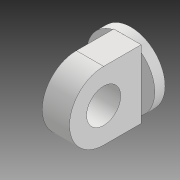
# Autodesk Inventor part: Link3
Saved by Autodesk Inventor 2020 (Build 240168000, 168)
## iProperties
Created: 2021-03-25
Part Number: Link3
Material: Generic
Document SubType Name: Modeling
Designer: DDeGo
Density: 1 g/cm^3
Appearance: Default
Author: DDeGo
Autodesk Inventor part; units mm, degrees
ref_plane "YZ Plane" through (0, 0, 0) normal (1, 0, 0) x (0, 1, 0)
ref_plane "XZ Plane" through (0, 0, 0) normal (0, 1, 0) x (-1, 0, 0)
ref_plane "XY Plane" through (0, 0, 0) normal (0, 0, 1) x (1, 0, 0)
sketch "Sketch1" plane through (0, 0, 0) normal (1, 0, 0) x (0, 1, 0)
  circle A0 centre (0, 0) radius 25
  arc A1 (50, 0) -> (-50, 0) centre (0, 0) ccw
  line L0 (50, 0) -> (-50, 0) construction
  line L1 (-50, 0) -> (-50, -55)
  line L2 (-50, -55) -> (50, -55)
  line L3 (50, -55) -> (50, 0)
  dimension "d0" = 50
  dimension "d1" = 100
  dimension "d4" = 55
  constraints: 8 end point, 2 centre point, 2 coincident, 2 parallel, 2 point on circle, 1 horizontal, 1 midpoint, 1 perpendicular
  measures "d0" diameter of A0
  measures "d1" diameter of A1
  measures "d4" distance from line of L2 point (0, 0)
extrude "Extrusion1" add sketch "Sketch1" along normal mid plane 40
sketch "Sketch2" plane through (-20, -50, -55) normal (0, 0, -1) x (-1, 0, 0)
  line L0 (-20, 50) -> (0, 50) construction
  circle A0 centre (0, 50) radius 50
  dimension "d5" = 100
  dimension "d9" = 20
  constraints: 2 end point, 1 centre point, 1 coincident, 1 horizontal
  measures "d5" diameter of A0
  measures "d9" distance of L0.start L0.end
extrude "Extrusion2" add sketch "Sketch2" along normal blind 15
body "Solid1"
